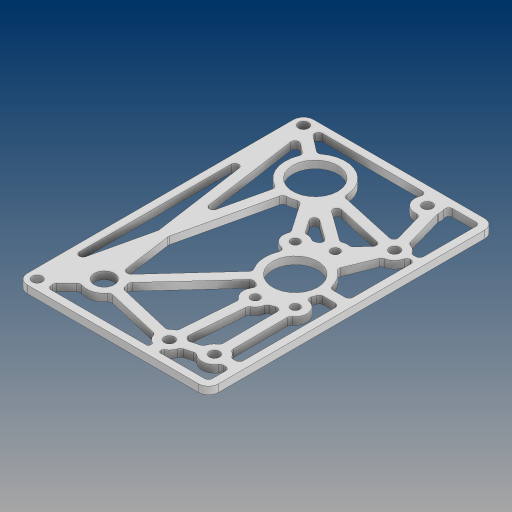
# Autodesk Inventor part: DragBarLinkage3 Bracket1
Saved by Autodesk Inventor 2024.3 (Build 283343000, 343)
## iProperties
Created: 2024-07-08
Part Number: DragBarLinkage3 Bracket1
Material: Generic
Document SubType Name: Modeling
Designer: Kenji
Density: 1 g/cm^3
Appearance: Default
Author: Kenji
Autodesk Inventor part; units mm, degrees
ref_plane "YZ Plane" through (0, 0, 0) normal (1, 0, 0) x (0, 1, 0)
ref_plane "XZ Plane" through (0, 0, 0) normal (0, 1, 0) x (-1, 0, 0)
ref_plane "XY Plane" through (0, 0, 0) normal (0, 0, 1) x (1, 0, 0)
sketch "Sketch1" plane through (0, 0, 0) normal (0, 1, 0) x (-1, 0, 0)
  circle A0 centre (-11.6078, -122.2341) radius 14.2875
  circle A1 centre (0, 0) radius 6.35
  line L0 (-88.9331, 22.86) -> (-88.9331, -149.2216) construction
  circle A2 centre (-11.6078, -122.2341) radius 26.9875 construction
  circle A3 centre (0, 0) radius 19.05 construction
  circle A4 centre (-53.9779, 12.7) radius 3.2512
  circle A5 centre (-62.1078, -142.8716) radius 3.2512
  circle A6 centre (-53.9779, 12.7) radius 6.35 construction
  circle A7 centre (-62.1078, -142.8716) radius 6.35 construction
  line L1 (-56.2297, -140.4694) -> (-36.5897, -132.4433) construction
  line L2 (-68.287, -144.3343) -> (-88.9331, -149.2216) construction
  line L3 (-47.7967, 11.2457) -> (-18.5436, 4.363) construction
  line L4 (-60.0756, 14.4723) -> (-88.9331, 22.86) construction
  line L5 (-88.9331, -32.1945) -> (-26.9571, -32.1945) construction
  line L6 (-26.9571, -32.1945) -> (-26.9571, -94.1705) construction
  line L7 (-26.9571, -94.1705) -> (-88.9331, -94.1705) construction
  line L8 (-88.9331, -94.1705) -> (-88.9331, -32.1945) construction
  circle A8 centre (-57.9451, -63.1825) radius 25.4 construction
  circle A9 centre (-57.9451, -88.5825) radius 2.794
  circle A10 centre (-39.9846, -81.143) radius 2.794
  circle A11 centre (-32.5451, -63.1825) radius 2.794 construction
  circle A12 centre (-39.9846, -45.222) radius 2.794 construction
  circle A13 centre (-57.9451, -37.7825) radius 2.794
  circle A14 centre (-75.9057, -45.222) radius 2.794
  circle A15 centre (-83.3451, -63.1825) radius 2.794 construction
  circle A16 centre (-75.9057, -81.143) radius 2.794 construction
  circle A17 centre (-57.9451, -63.1825) radius 14.2875
  circle A18 centre (-57.9451, -63.1825) radius 22.86 construction
  circle A19 centre (0, 0) radius 22.86 construction
  line L9 (-88.9331, 22.86) -> (22.86, 22.86) construction
  line L10 (22.86, 22.86) -> (22.86, -149.2216) construction
  line L11 (-88.9331, -149.2216) -> (22.86, -149.2216) construction
  line L12 (-93.7083, -147.6341) -> (-93.7083, 21.2725)
  circle A20 centre (21.2725, 21.2725) radius 3.2512
  circle A21 centre (21.2725, 21.2725) radius 6.35 construction
  circle A22 centre (21.2725, -147.6341) radius 3.2512
  circle A23 centre (21.2725, -147.6341) radius 6.35 construction
  line L13 (16.2473, -143.7521) -> (9.7494, -138.7325) construction
  line L14 (16.7824, 16.7824) -> (16.1645, 16.1645) construction
  line L15 (27.6225, 21.2725) -> (27.6225, -147.6341)
  line L16 (21.2725, -153.9841) -> (-87.3583, -153.9841)
  line L17 (21.2725, 27.6225) -> (-87.3583, 27.6225)
  arc A24 (27.6225, 21.2725) -> (21.2725, 27.6225) centre (21.2725, 21.2725) ccw
  arc A25 (21.2725, -153.9841) -> (27.6225, -147.6341) centre (21.2725, -147.6341) ccw
  arc A26 (-87.3583, 27.6225) -> (-93.7083, 21.2725) centre (-87.3583, 21.2725) ccw
  arc A27 (-93.7083, -147.6341) -> (-87.3583, -153.9841) centre (-87.3583, -147.6341) ccw
  circle A28 centre (-76.2331, -107.95) radius 3.2512
  circle A29 centre (-76.2331, 6.35) radius 3.2512
  line L18 (-11.6078, -122.2341) -> (-11.6078, 16.1596) construction
  line L19 (-11.6078, 0) -> (0, 0) construction
  circle A30 centre (-57.9451, -63.1825) radius 19.9136 construction
  circle A31 centre (-11.6078, -122.2341) radius 19.9136 construction
  line L20 (-73.6113, -75.4757) -> (-27.274, -134.5272) construction
  point P0 (0, 19.05)
  point P1 (-11.6078, -149.2216)
  point P2 (-62.1078, -149.2216)
  point P3 (-53.9779, 19.05)
  point P4 (-26.9571, -63.1825)
  point P5 (-57.9451, -32.1945)
  point P6 (0, -63.1825)
  point P7 (0, 22.86)
  point P8 (-93.7083, 27.6225)
  point P9 (-93.7083, -153.9841)
  point P10 (-33.0429, 27.6225)
  point P11 (22.86, -63.1825)
  point P12 (-53.9779, 6.35)
  dimension "d19" = 50.8
  dimension "d289" = 39.8272
  dimension "d290" = 39.8272
  dimension "d1" = 28.575
  dimension "d2" = 12.7
  dimension "d4" = 12.7
  dimension "d5" = 12.7
  dimension "d6" = 6.5024
  dimension "d7" = 6.5024
  dimension "d8" = 12.7
  dimension "d9" = 12.7
  dimension "d17" = 61.976
  dimension "d18" = 61.976
  dimension "d20" = 5.588
  dimension "d23" = 360
  dimension "d25" = 28.575
  dimension "d26" = 45.72
  dimension "d27" = 45.72
  dimension "d31" = 4.7752
  dimension "d32" = 6.5024
  dimension "d33" = 12.7
  dimension "d34" = 6.5024
  dimension "d35" = 12.7
  dimension "d38" = 4.7625
  dimension "d39" = 4.7625
  dimension "d40" = 4.7625
  dimension "d41" = 6.35
  dimension "d42" = 6.35
  dimension "d134" = 6.5024
  dimension "d135" = 6.5024
  dimension "d136" = 12.7
  dimension "d162" = 11.6078
  dimension "d163" = 86.0425
  dimension "d165" = 172.0816
  dimension "d166" = 15.3493
  dimension "d167" = 114.3
  constraints: 44 end point, 29 centre point, 28 point on circle, 18 point on line, 11 tangent, 11 vertical alignment, 10 coincident, 8 horizontal alignment, 5 perpendicular, 3 concentric, 3 horizontal, 3 midpoint, 2 equal length, 2 parallel, 1 collinear, 1 vertical, 28 other
  measures "d1" diameter of A0
  measures "d2" diameter of A1
  measures "d4" radial gap between concentric circles of A0 A2
  measures "d5" radial gap between concentric circles of A1 A3
  measures "d6" diameter of A4
  measures "d7" diameter of A5
  measures "d8" diameter of A6
  measures "d9" diameter of A7
  measures "d17" distance of L6.end L7.end
  measures "d18" distance of L5.end L6.end
  measures "d20" diameter of A9
  measures "d25" diameter of A17
  measures "d26" diameter of A18
  measures "d27" diameter of A19
  measures "d31" distance between parallel lines of L12 L0
  measures "d32" diameter of A20
  measures "d33" diameter of A21
  measures "d34" diameter of A22
  measures "d35" diameter of A23
  measures "d38" distance between parallel lines of L10 L15
  measures "d39" distance between parallel lines of L16 L11
  measures "d40" distance from line of point (-33.043, 27.623) L9
  measures "d41" radius of A26
  measures "d42" radius of A27
  measures "d134" diameter of A28
  measures "d135" diameter of A29
  measures "d136" distance from line of L0 A29.centre
  measures "d162" distance of L19.start L19.end
  measures "d163" distance of L9.end point (22.86, -63.183)
  measures "d165" distance of L9.end L10.end
  measures "d166" distance between parallel lines of L6 L18
  measures "d167" distance of A28.centre A29.centre
extrude "Extrusion2" add sketch "Sketch1" along normal blind 4.7625 contours L12 A26 L17 A24 L15 A25 L16 A27 | A28 | A29
extrude "Extrusion5" cut sketch "Sketch1" along normal blind 25.4 contours A28 | A29
sketch "Sketch6" plane through (0, 4.7625, 0) normal (0, 1, 0) x (1, 0, 0)
  circle A0 centre (76.2331, -6.35) radius 3.2512 projected
  circle A1 centre (76.2331, 107.95) radius 3.2512 projected
  line L0 (-27.6225, 147.6341) -> (-27.6225, -21.2725) projected
  arc A2 (-27.6225, -21.2725) -> (-21.2725, -27.6225) centre (-21.2725, -21.2725) ccw projected
  line L1 (-21.2725, -27.6225) -> (87.3583, -27.6225) projected
  arc A3 (87.3583, -27.6225) -> (93.7083, -21.2725) centre (87.3583, -21.2725) ccw projected
  line L2 (93.7083, -21.2725) -> (93.7083, 147.6341) projected
  arc A4 (93.7083, 147.6341) -> (87.3583, 153.9841) centre (87.3583, 147.6341) ccw projected
  line L3 (87.3583, 153.9841) -> (-21.2725, 153.9841) projected
  arc A5 (-21.2725, 153.9841) -> (-27.6225, 147.6341) centre (-21.2725, 147.6341) ccw projected
  circle A6 centre (57.9451, 63.1825) radius 14.2875 projected
  circle A7 centre (11.6078, 122.2341) radius 14.2875 projected
  circle A8 centre (0, 0) radius 6.35 projected
  circle A9 centre (53.9779, -12.7) radius 3.2512 projected
  circle A10 centre (62.1078, 142.8716) radius 3.2512 projected
  circle A11 centre (57.9451, 88.5825) radius 2.794 projected
  circle A12 centre (39.9846, 81.143) radius 2.794 projected
  circle A13 centre (57.9451, 37.7825) radius 2.794 projected
  circle A14 centre (75.9057, 45.222) radius 2.794 projected
  circle A15 centre (-21.2725, 147.6341) radius 3.2512 projected
  circle A16 centre (-21.2725, -21.2725) radius 3.2512 projected
  circle A17 centre (0, 0) radius 11.1252 construction
  circle A18 centre (-21.2725, -21.2725) radius 8.0137 construction
  circle A19 centre (11.6078, 122.2341) radius 19.05 construction
  circle A20 centre (57.9451, 63.1825) radius 19.05 construction
  circle A21 centre (39.9846, 81.143) radius 7.5565 construction
  circle A22 centre (57.9451, 37.7825) radius 7.5565 construction
  circle A23 centre (75.9057, 45.222) radius 7.5565 construction
  circle A24 centre (57.9451, 88.5825) radius 7.5565 construction
  circle A25 centre (76.2331, 107.95) radius 8.0137 construction
  circle A26 centre (62.1078, 142.8716) radius 8.0137 construction
  circle A27 centre (-21.2725, 147.6341) radius 8.0137 construction
  circle A28 centre (53.9779, -12.7) radius 8.0137 construction
  circle A29 centre (76.2331, -6.35) radius 8.0137 construction
  line L4 (-15.606, -15.606) -> (-7.8667, -7.8667) construction
  line L5 (7.5195, 8.1992) -> (45.0692, 49.1428) construction
  line L6 (35.6906, 87.3609) -> (22.433, 106.5587) construction
  line L7 (-3.4678, 133.88) -> (-14.9307, 142.735) construction
  line L8 (27.0219, 111.0399) -> (51.8309, 93.0228) construction
  line L9 (57.3531, 30.2492) -> (54.6057, -4.7109) construction
  line L10 (46.1772, -10.8646) -> (10.8295, -2.548) construction
  line L11 (61.6841, -10.5012) -> (68.527, -8.5488) construction
  line L12 (76.1823, 1.6635) -> (75.9536, 37.6656) construction
  line L13 (63.1331, 94.0767) -> (70.7313, 102.1234) construction
  line L14 (73.2026, 100.5314) -> (65.1493, 80.8178) construction
  line L15 (68.4083, 109.6795) -> (30.2089, 118.1227) construction
  line L16 (74.0344, 115.6562) -> (67.8609, 137.2929) construction
  line L17 (-22.8473, -21.2725) -> (-22.8473, 147.6341) construction
  arc A30 (-21.2725, 149.2089) -> (-22.8473, 147.6341) centre (-21.2725, 147.6341) ccw construction
  line L18 (-10.9265, 149.2089) -> (86.5709, 149.2089) construction
  arc A31 (88.9331, 147.6341) -> (87.3583, 149.2089) centre (87.3583, 147.6341) ccw construction
  line L19 (88.9331, -11.8872) -> (88.9331, -21.2725) construction
  arc A32 (87.3583, -22.8473) -> (88.9331, -21.2725) centre (87.3583, -21.2725) ccw construction
  line L20 (87.3583, -22.8473) -> (-10.9265, -22.8473) construction
  arc A33 (-22.8473, -21.2725) -> (-21.2725, -22.8473) centre (-21.2725, -21.2725) ccw construction
  line L21 (76.9951, 63.1825) -> (88.9331, 63.1825) construction
  line L22 (46.9659, 84.0348) -> (50.9638, 85.6908) construction
  line L23 (64.9264, 40.6742) -> (68.9244, 42.3302) construction
  line L24 (-19.4828, -13.4612) -> (7.3533, 103.6652) construction
  line L25 (-20.1296, 139.7023) -> (-6.3312, 43.9392) construction
  line L26 (-18.1826, 6.43) -> (-9.6563, 43.6428)
  line L27 (-18.147, 103.6805) -> (-9.6208, 44.5073)
  line L28 (-22.8473, 6.9575) -> (-22.8473, 103.3436)
  arc A34 (-22.8473, 6.9575) -> (-18.1826, 6.43) centre (-20.4851, 6.9575) ccw
  arc A35 (-18.147, 103.6805) -> (-22.8473, 103.3436) centre (-20.4851, 103.3436) ccw
  arc A36 (-9.6563, 43.6428) -> (-9.6208, 44.5073) centre (-11.9589, 44.1704) ccw
  line L29 (-16.181, 134.5609) -> (-7.4279, 73.8134)
  line L30 (-3.006, 44.2355) -> (10.0832, 101.3636)
  line L31 (-2.7873, 73.6227) -> (3.8936, 102.7817)
  line L32 (-6.7018, 132.3662) -> (-12.3989, 136.7672)
  line L33 (-6.3312, 43.9392) -> (-1.5866, 11.0115) construction
  line L34 (1.3886, 12.6254) -> (-3.0415, 43.3711)
  line L35 (5.9725, 11.2098) -> (41.625, 50.0846)
  line L36 (32.6958, 86.1103) -> (20.7488, 103.4101)
  arc A37 (12.2999, 103.1967) -> (18.0111, 104.2925) centre (11.6078, 122.2341) ccw
  arc A38 (32.9509, 83.9046) -> (38.6015, 73.7142) centre (39.9846, 81.143) ccw
  arc A39 (40.3509, 70.4862) -> (41.8765, 52.9501) centre (57.9451, 63.1825) ccw
  arc A40 (3.4905, 10.5635) -> (3.074, 10.6921) centre (0, 0) ccw
  arc A41 (1.3886, 12.6254) -> (3.074, 10.6921) centre (3.7267, 12.9623) ccw
  arc A42 (3.4905, 10.5635) -> (5.9725, 11.2098) centre (4.2316, 12.8064) ccw
  arc A43 (-3.006, 44.2355) -> (-3.0415, 43.3711) centre (-0.7035, 43.7079) ccw
  arc A44 (41.625, 50.0846) -> (41.8765, 52.9501) centre (39.884, 51.6813) ccw
  arc A45 (40.3509, 70.4862) -> (38.6015, 73.7142) centre (38.1692, 71.3919) ccw
  arc A46 (32.9509, 83.9046) -> (32.6958, 86.1103) centre (30.7521, 84.768) ccw
  arc A47 (20.7488, 103.4101) -> (18.0111, 104.2925) centre (18.8051, 102.0677) ccw
  arc A48 (12.2999, 103.1967) -> (10.0832, 101.3636) centre (12.3857, 100.836) ccw
  arc A49 (-7.4279, 73.8134) -> (-2.7873, 73.6227) centre (-5.0899, 74.1502) ccw
  arc A50 (-12.3989, 136.7672) -> (-16.181, 134.5609) centre (-13.843, 134.8978) ccw
  arc A51 (-5.9667, 129.5853) -> (2.6961, 105.3971) centre (11.6078, 122.2341) ccw
  arc A52 (3.8936, 102.7817) -> (2.6961, 105.3971) centre (1.5911, 103.3093) ccw
  arc A53 (-5.9667, 129.5853) -> (-6.7018, 132.3662) centre (-8.1459, 130.4968) ccw
  line L37 (-12.8227, -17.3128) -> (-6.4512, -10.9413)
  line L38 (44.7091, -13.7809) -> (11.2443, -5.9073)
  line L39 (53.9779, -20.7137) -> (53.9779, -22.8473) construction
  line L40 (84.2468, -6.35) -> (88.9331, -6.35) construction
  line L41 (-13.4151, -22.8473) -> (49.6218, -22.8473)
  arc A54 (46.4014, -15.3108) -> (50.1814, -19.7573) centre (53.9779, -12.7) ccw
  arc A55 (-3.9435, -10.4028) -> (8.8287, -6.7694) centre (0, 0) ccw
  arc A56 (-13.2819, -20.6644) -> (-13.4563, -19.5043) centre (-21.2725, -21.2725) ccw
  arc A57 (-12.8227, -17.3128) -> (-13.4563, -19.5043) centre (-11.1523, -18.9831) ccw
  arc A58 (-13.2819, -20.6644) -> (-10.9265, -22.8473) centre (-10.9265, -20.4851) ccw
  arc A59 (-3.9435, -10.4028) -> (-6.4512, -10.9413) centre (-4.7809, -12.6116) ccw
  arc A60 (11.2443, -5.9073) -> (8.8287, -6.7694) centre (10.7033, -8.2067) ccw
  arc A61 (46.4014, -15.3108) -> (44.7091, -13.7809) centre (44.1681, -16.0803) ccw
  circle A62 centre (49.6218, -21.6662) radius 1.1811 construction
  arc A63 (48.5235, -21.2318) -> (50.7201, -21.2318) centre (49.6218, -20.7975) ccw construction
  line L42 (50.8029, -20.7975) -> (50.8029, -21.6662)
  arc A64 (50.8029, -20.7975) -> (50.1814, -19.7573) centre (49.6218, -20.7975) ccw construction
  arc A65 (49.6218, -22.8473) -> (50.8029, -21.6662) centre (49.6218, -21.6662) ccw
  arc A66 (50.8029, -20.7975) -> (50.1814, -19.7573) centre (49.6218, -20.7975) ccw
  line L43 (46.1634, -7.5997) -> (12.6986, 0.2739)
  line L44 (10.6524, 6.9178) -> (46.3049, 45.7927)
  line L45 (54.1352, 29.8273) -> (51.5001, -3.7033)
  arc A67 (50.2454, -5.6086) -> (48.3603, -6.9849) centre (53.9779, -12.7) ccw
  arc A68 (49.1379, 46.2907) -> (50.6686, 45.577) centre (57.9451, 63.1825) ccw
  arc A69 (51.7142, 42.0575) -> (53.2485, 31.8629) centre (57.9451, 37.7825) ccw
  arc A70 (10.9208, 2.1227) -> (10.2228, 4.3892) centre (0, 0) ccw
  arc A71 (10.6524, 6.9178) -> (10.2228, 4.3892) centre (12.3933, 5.3212) ccw
  arc A72 (10.9208, 2.1227) -> (12.6986, 0.2739) centre (13.2396, 2.5734) ccw
  arc A73 (46.1634, -7.5997) -> (48.3603, -6.9849) centre (46.7044, -5.3003) ccw
  arc A74 (50.2454, -5.6086) -> (51.5001, -3.7033) centre (49.1452, -3.5183) ccw
  arc A75 (49.1379, 46.2907) -> (46.3049, 45.7927) centre (48.0458, 44.1961) ccw
  arc A76 (51.7142, 42.0575) -> (50.6686, 45.577) centre (49.7663, 43.3939) ccw
  arc A77 (54.1352, 29.8273) -> (53.2485, 31.8629) centre (51.7802, 30.0124) ccw
  line L46 (37.9209, 89.7187) -> (32.6443, 97.3594)
  line L47 (35.9762, 100.6131) -> (48.0773, 91.8249)
  line L48 (46.3724, 87.2255) -> (47.5932, 87.7312)
  arc A78 (35.9762, 100.6131) -> (32.6443, 97.3594) centre (34.5881, 98.7018) ccw
  arc A79 (50.5311, 90.0429) -> (50.395, 88.8917) centre (57.9451, 88.5825) ccw
  arc A80 (44.1624, 87.4396) -> (39.8933, 88.699) centre (39.9846, 81.143) ccw
  arc A81 (37.9209, 89.7187) -> (39.8933, 88.699) centre (39.8647, 91.061) ccw
  arc A82 (44.1624, 87.4396) -> (46.3724, 87.2255) centre (45.4684, 89.4079) ccw
  arc A83 (47.5932, 87.7312) -> (48.0773, 91.8249) centre (46.6892, 89.9136) ccw
  line L49 (60.4657, 29.3298) -> (57.8306, -4.2008)
  line L50 (61.5449, -7.2392) -> (66.9239, -5.7045)
  line L51 (73.0025, 2.4046) -> (72.783, 36.9717)
  line L52 (66.763, 37.9984) -> (69.5169, 39.1391)
  arc A84 (59.3216, -6.728) -> (58.7723, -6.2787) centre (53.9779, -12.7) ccw
  arc A85 (61.6595, 31.2019) -> (65.3516, 36.2843) centre (57.9451, 37.7825) ccw
  arc A86 (70.7855, 39.6646) -> (72.7743, 38.3448) centre (75.9057, 45.222) ccw
  arc A87 (71.9136, 0.3999) -> (68.5427, -4.097) centre (76.2331, -6.35) ccw
  arc A88 (57.8306, -4.2008) -> (58.7723, -6.2787) centre (60.1856, -4.3859) ccw
  arc A89 (59.3216, -6.728) -> (61.5449, -7.2392) centre (60.8968, -4.9677) ccw
  arc A90 (61.6595, 31.2019) -> (60.4657, 29.3298) centre (62.8206, 29.1448) ccw
  arc A91 (66.763, 37.9984) -> (65.3516, 36.2843) centre (67.6669, 35.816) ccw
  arc A92 (72.783, 36.9717) -> (69.5169, 39.1391) centre (70.4208, 36.9567) ccw
  arc A93 (66.9239, -5.7045) -> (68.5427, -4.097) centre (66.2757, -3.4329) ccw
  arc A94 (71.9136, 0.3999) -> (73.0025, 2.4046) centre (70.6403, 2.3896) ccw
  line L53 (63.2872, -13.3455) -> (68.6662, -11.8108)
  line L54 (85.008, -9.525) -> (86.5709, -9.525)
  line L55 (88.9331, -9.525) -> (88.9331, -20.4851)
  arc A95 (70.8894, -12.322) -> (83.0103, -10.6266) centre (76.2331, -6.35) ccw
  arc A96 (63.2872, -13.3455) -> (61.6684, -14.953) centre (63.9353, -15.6171) ccw
  arc A97 (70.8894, -12.322) -> (68.6662, -11.8108) centre (69.3143, -14.0823) ccw
  arc A98 (85.008, -9.525) -> (83.0103, -10.6266) centre (85.008, -11.8872) ccw
  arc A99 (88.9331, -11.8872) -> (86.5709, -9.525) centre (86.5709, -11.8872) ccw
  arc A100 (86.5709, -22.8473) -> (88.9331, -20.4851) centre (86.5709, -20.4851) ccw
  circle A101 centre (58.334, -20.7975) radius 1.1811 construction
  circle A102 centre (58.334, -21.6662) radius 1.1811 construction
  line L56 (57.1529, -20.7975) -> (57.1529, -21.6662)
  arc A103 (57.7745, -19.7573) -> (61.6684, -14.953) centre (53.9779, -12.7) ccw
  line L57 (58.334, -22.8473) -> (86.5709, -22.8473)
  arc A104 (57.1529, -21.6662) -> (58.334, -22.8473) centre (58.334, -21.6662) ccw
  arc A105 (57.7745, -19.7573) -> (57.1529, -20.7975) centre (58.334, -20.7975) ccw
  line L58 (85.008, -3.175) -> (86.5709, -3.175)
  line L59 (79.3524, 2.4449) -> (79.1328, 37.0131)
  line L60 (78.629, 60.0075) -> (86.5709, 60.0075)
  line L61 (88.9331, -0.8128) -> (88.9331, 57.6453)
  arc A106 (80.1639, 38.9795) -> (77.2887, 52.6508) centre (75.9057, 45.222) ccw
  arc A107 (75.5394, 55.8788) -> (76.3471, 58.2562) centre (57.9451, 63.1825) ccw
  arc A108 (83.0103, -2.0734) -> (80.4666, 0.4542) centre (76.2331, -6.35) ccw
  arc A109 (79.3524, 2.4449) -> (80.4666, 0.4542) centre (81.7145, 2.4599) ccw
  arc A110 (83.0103, -2.0734) -> (85.008, -3.175) centre (85.008, -0.8128) ccw
  arc A111 (86.5709, -3.175) -> (88.9331, -0.8128) centre (86.5709, -0.8128) ccw
  arc A112 (80.1639, 38.9795) -> (79.1328, 37.0131) centre (81.495, 37.0281) ccw
  arc A113 (75.5394, 55.8788) -> (77.2887, 52.6508) centre (77.7211, 54.9731) ccw
  arc A114 (78.629, 60.0075) -> (76.3471, 58.2562) centre (78.629, 57.6453) ccw
  arc A115 (88.9331, 57.6453) -> (86.5709, 60.0075) centre (86.5709, 57.6453) ccw
  line L62 (75.8539, 98.6261) -> (68.7064, 81.1296)
  line L63 (78.629, 66.3575) -> (86.5709, 66.3575)
  line L64 (76.8787, 117.2593) -> (70.1293, 140.9144)
  line L65 (84.2468, 107.95) -> (93.7083, 107.95) construction
  line L66 (88.9331, 68.7197) -> (88.9331, 105.5878)
  line L67 (86.3366, 107.95) -> (86.5709, 107.95)
  arc A116 (77.6292, 100.0588) -> (84.0364, 106.1256) centre (76.2331, 107.95) ccw
  arc A117 (76.3471, 68.1088) -> (69.4648, 78.3549) centre (57.9451, 63.1825) ccw
  arc A118 (68.7064, 81.1296) -> (69.4648, 78.3549) centre (70.8932, 80.2362) ccw
  arc A119 (76.3471, 68.1088) -> (78.629, 66.3575) centre (78.629, 68.7197) ccw
  arc A120 (86.5709, 66.3575) -> (88.9331, 68.7197) centre (86.5709, 68.7197) ccw
  arc A121 (77.6292, 100.0588) -> (75.8539, 98.6261) centre (78.0407, 97.7328) ccw
  arc A122 (86.3366, 107.95) -> (84.0364, 106.1256) centre (86.3366, 105.5878) ccw
  arc A123 (88.9331, 105.5878) -> (86.5709, 107.95) centre (86.5709, 105.5878) ccw
  line L68 (85.008, 111.125) -> (86.5709, 111.125)
  line L69 (88.9331, 113.4872) -> (88.9331, 146.8467)
  arc A124 (83.0103, 112.2266) -> (78.4861, 115.6405) centre (76.2331, 107.95) ccw
  arc A125 (70.0575, 141.8605) -> (69.5101, 145.9417) centre (62.1078, 142.8716) ccw
  line L70 (71.6921, 149.2089) -> (88.9331, 149.2089)
  arc A126 (76.8787, 117.2593) -> (78.4861, 115.6405) centre (79.1502, 117.9074) ccw
  arc A127 (83.0103, 112.2266) -> (85.008, 111.125) centre (85.008, 113.4872) ccw
  arc A128 (86.5709, 111.125) -> (88.9331, 113.4872) centre (86.5709, 113.4872) ccw
  arc A129 (88.9331, 146.8467) -> (86.5709, 149.2089) centre (86.5709, 146.8467) ccw
  arc A130 (71.6921, 149.2089) -> (69.5101, 145.9417) centre (71.6921, 146.8467) ccw
  arc A131 (70.0575, 141.8605) -> (70.1293, 140.9144) centre (72.4008, 141.5625) ccw
  line L71 (34.9904, 109.1768) -> (53.1523, 95.9872)
  line L72 (66.0121, 106.9575) -> (36.8883, 113.3947)
  line L73 (61.2865, 96.7456) -> (67.2198, 103.0292)
  arc A132 (28.672, 113.7655) -> (29.2635, 115.08) centre (11.6078, 122.2341) ccw
  arc A133 (59.1822, 96.037) -> (55.3512, 95.6798) centre (57.9451, 88.5825) ccw
  arc A134 (68.3634, 106.4378) -> (68.8731, 104.78) centre (76.2331, 107.95) ccw
  arc A135 (36.8883, 113.3947) -> (34.9904, 109.1768) centre (36.3785, 111.0882) ccw
  arc A136 (53.1523, 95.9872) -> (55.3512, 95.6798) centre (54.5403, 97.8985) ccw
  arc A137 (59.1822, 96.037) -> (61.2865, 96.7456) centre (59.569, 98.3674) ccw
  arc A138 (67.2198, 103.0292) -> (66.0121, 106.9575) centre (65.5023, 104.651) ccw
  line L74 (-2.8198, 137.3914) -> (-12.3873, 144.7823)
  line L75 (67.8506, 113.0544) -> (32.4894, 120.8703)
  line L76 (70.632, 116.0091) -> (65.7182, 133.2306)
  line L77 (-13.4151, 149.2089) -> (52.5236, 149.2089)
  arc A139 (30.6393, 123.0728) -> (0.0566, 137.3824) centre (11.6078, 122.2341) ccw
  arc A140 (-13.2948, 146.8753) -> (-13.2819, 147.0259) centre (-21.2725, 147.6341) ccw
  arc A141 (54.7055, 145.9417) -> (63.1419, 134.9249) centre (62.1078, 142.8716) ccw
  arc A142 (71.1612, 114.1544) -> (69.7339, 112.6382) centre (76.2331, 107.95) ccw
  arc A143 (-13.2948, 146.8753) -> (-12.3873, 144.7823) centre (-10.9432, 146.6517) ccw
  arc A144 (-10.9265, 149.2089) -> (-13.2819, 147.0259) centre (-10.9265, 146.8467) ccw
  arc A145 (-2.8198, 137.3914) -> (0.0566, 137.3824) centre (-1.3757, 139.2608) ccw
  arc A146 (30.6393, 123.0728) -> (32.4894, 120.8703) centre (32.9992, 123.1768) ccw
  arc A147 (67.8506, 113.0544) -> (70.632, 116.0091) centre (68.3604, 115.3609) ccw
  arc A148 (65.7182, 133.2306) -> (63.1419, 134.9249) centre (63.4467, 132.5824) ccw
  arc A149 (54.7055, 145.9417) -> (52.5236, 149.2089) centre (52.5236, 146.8467) ccw
  point P0 (-22.8473, 63.1808)
  point P1 (-22.724, -13.3914)
  point P2 (-22.8473, 136.3009)
  point P3 (-22.8473, -13.4151)
  point P4 (-3.1043, 43.8066)
  point P5 (10.5076, 103.2159)
  point P6 (4.318, 104.634)
  point P7 (-5.198, 131.2045)
  point P8 (1.6219, 11.0063)
  point P9 (4.8669, 10.0042)
  point P10 (42.9094, 51.4852)
  point P11 (33.4755, 84.9812)
  point P12 (19.669, 104.9737)
  point P13 (-13.8246, -18.3147)
  point P14 (-5.2945, -9.7846)
  point P15 (46.0884, -14.1054)
  point P16 (9.652, -5.5326)
  point P17 (47.5428, -7.9242)
  point P18 (11.1063, 0.6486)
  point P19 (9.5468, 5.7122)
  point P20 (47.5893, 47.1932)
  point P21 (54.2427, 31.1952)
  point P22 (51.3891, -5.116)
  point P23 (38.7006, 88.5896)
  point P24 (24.8941, 108.5821)
  point P25 (24.9406, 108.6275)
  point P26 (45.1048, 86.7004)
  point P27 (60.5732, 30.6977)
  point P28 (57.7196, -5.6135)
  point P29 (60.1823, -7.628)
  point P30 (68.2865, -5.3157)
  point P31 (73.0115, 0.9876)
  point P32 (65.4953, 37.4733)
  point P33 (61.9246, -13.7343)
  point P34 (70.0288, -11.422)
  point P35 (83.591, -9.525)
  point P36 (83.591, -3.175)
  point P37 (79.3614, 1.0279)
  point P38 (79.1241, 38.3852)
  point P39 (76.7287, 60.0075)
  point P40 (76.3898, 99.9378)
  point P41 (67.9878, 79.3704)
  point P42 (76.7287, 66.3575)
  point P43 (77.2675, 115.8967)
  point P44 (69.9874, 141.4116)
  point P45 (88.9331, 107.95)
  point P46 (83.591, 111.125)
  point P47 (67.0127, 149.2089)
  point P48 (54.2625, 95.1809)
  point P49 (60.3444, 95.748)
  point P50 (-1.316, 136.2297)
  point P51 (-13.5087, 145.6485)
  point P52 (30.6339, 121.2804)
  point P53 (65.0897, 135.4333)
  point P54 (57.2029, 149.2089)
  point P55 (57.7745, -19.7573)
  dimension "d199" = 4.7752
  dimension "d200" = 4.7625
  dimension "d201" = 4.7625
  dimension "d202" = 4.7625
  dimension "d203" = 4.7625
  dimension "d204" = 4.7752
  dimension "d205" = 4.7752
  dimension "d206" = 4.7752
  dimension "d207" = 4.7752
  dimension "d208" = 4.7752
  dimension "d209" = 3.175
  dimension "d210" = 3.175
  dimension "d211" = 2.3622
  dimension "d212" = 2.3622
  dimension "d213" = 2.3622
  dimension "d217" = 3.175
  dimension "d218" = 3.175
  dimension "d219" = 3.175
  dimension "d220" = 3.175
  dimension "d223" = 3.175
  dimension "d224" = 3.175
  dimension "d225" = 3.175
  dimension "d226" = 2.3622
  dimension "d227" = 2.3622
  dimension "d228" = 2.3622
  dimension "d229" = 2.3622
  dimension "d230" = 3.175
  dimension "d231" = 3.175
  dimension "d233" = 2.3622
  dimension "d234" = 2.3622
  dimension "d235" = 2.3622
  dimension "d236" = 3.175
  dimension "d237" = 3.175
  dimension "d238" = 3.175
  dimension "d239" = 3.175
  dimension "d240" = 2.3622
  dimension "d241" = 3.175
  dimension "d243" = 3.175
  dimension "d244" = 3.175
  dimension "d245" = 2.3622
  dimension "d246" = 2.3622
  dimension "d247" = 3.175
  dimension "d248" = 3.175
  dimension "d249" = 3.175
  dimension "d250" = 3.175
  dimension "d251" = 2.3622
  dimension "d252" = 2.3622
  dimension "d253" = 2.3622
  dimension "d254" = 3.175
  dimension "d256" = 3.175
  dimension "d257" = 2.3622
  dimension "d258" = 2.3622
  dimension "d259" = 2.3622
  dimension "d260" = 2.3622
  dimension "d261" = 3.175
  dimension "d262" = 4.7625
  dimension "d263" = 3.175
  dimension "d264" = 3.175
  dimension "d265" = 3.175
  dimension "d266" = 4.7752
  dimension "d267" = 2.3622
  dimension "d268" = 2.3622
  dimension "d269" = 3.175
  dimension "d270" = 3.175
  constraints: 321 point on circle, 156 tangent, 148 end point, 126 centre point, 126 point on line, 54 equal radius, 16 concentric, 8 parallel, 5 collinear, 5 perpendicular, 2 horizontal alignment, 2 vertical, 2 vertical alignment, 1 coincident, 1 horizontal, 1 midpoint, 119 other
  measures "d200" radial gap between concentric circles of A16 A18
  measures "d204" distance between parallel lines of L18 L3
  measures "d205" distance between parallel lines of L17 L0
  measures "d206" distance between parallel lines of L1 L20
  measures "d207" distance between parallel lines of L2 L19
  measures "d208" distance of L2.start L19.end
  measures "d209" distance between parallel lines of L25 L27
  measures "d210" distance between parallel lines of L24 L26
  measures "d211" radius of A34
  measures "d212" radius of A35
  measures "d213" radius of A36
  measures "d217" distance between parallel lines of L29 L25
  measures "d218" distance between parallel lines of L7 L32
  measures "d219" distance between parallel lines of L24 L31
  measures "d220" distance between parallel lines of L30 L24
  measures "d223" distance between parallel lines of L34 L33
  measures "d224" distance between parallel lines of L5 L35
  measures "d225" distance between parallel lines of L6 L36
  measures "d226" radius of A41
  measures "d227" radius of A43
  measures "d228" radius of A49
  measures "d229" radius of A52
  measures "d230" distance between parallel lines of L10 L38
  measures "d231" distance between parallel lines of L37 L4
  measures "d233" radius of A57
  measures "d234" diameter of A62
  measures "d235" diameter of A63
  measures "d236" distance between parallel lines of L39 L42
  measures "d237" distance between parallel lines of L10 L43
  measures "d238" distance between parallel lines of L44 L5
  measures "d239" distance between parallel lines of L9 L45
  measures "d240" radius of A71
  measures "d241" distance between parallel lines of L8 L47
  measures "d243" distance between parallel lines of L22 L48
  measures "d244" distance between parallel lines of L6 L46
  measures "d245" radius of A78
  measures "d246" radius of A81
  measures "d247" distance between parallel lines of L52 L23
  measures "d248" distance between parallel lines of L49 L9
  measures "d249" distance between parallel lines of L11 L50
  measures "d250" distance between parallel lines of L12 L51
  measures "d251" radius of A88
  measures "d252" radius of A92
  measures "d253" radius of A93
  measures "d254" distance between parallel lines of L53 L11
  measures "d256" distance between parallel lines of L40 L54
  measures "d257" radius of A96
  measures "d258" radius of A100
  measures "d259" diameter of A101
  measures "d260" diameter of A102
  measures "d261" distance between parallel lines of L39 L56
  measures "d262" radial gap between concentric circles of A9 A103
  measures "d263" distance between parallel lines of L59 L12
  measures "d264" distance between parallel lines of L40 L58
  measures "d265" distance between parallel lines of L21 L60
  measures "d266" distance between parallel lines of L2 L61
  measures "d267" radius of A109
  measures "d268" radius of A115
  measures "d269" distance between parallel lines of L21 L63
  measures "d270" distance between parallel lines of L14 L62
extrude "Extrusion6" cut sketch "Sketch6" against normal blind 25.4 contours A34 L28 A35 L27 A36 L26 | A50 L32 A53 A51 A52 L31 A49 L29 | L30 A48 A37 A47 L36 A46 A38 A45 A39 A44 L35 A42 A40 A41 L34 A43 | L37 A59 A55 A60 L38 A61 A54 A66 L42 A65 L41 A58 A56 A57 | L43 A72 A70 A71 L44 A75 A68 A76 A69 A77 L45 A74 A67 A73 | L46 A78 L47 A83 L48 A82 A80 A81 | A90 A85 A91 L52 A92 L51 A94 A87 A93 L50 A89 A84 A88 L49 | L53 A97 A95 A98 L54 A99 L55 A100 L57 A104 L56 A105 A103 A96 | A110 A108 A109 L59 A112 A106 A113 A107 A114 L60 A115 L61 A111 L58 | A121 A116 A122 L67 A123 L66 A120 L63 A119 A117 A118 L62 | L64 A131 A125 A130 L70 A129 L69 A128 L68 A127 A124 A126 | A135 L72 A138 L73 A137 A133 A136 L71 | L74 A143 A140 A144 L77 A149 A141 A148 L76 A147 L75 A146 A139 A145
body "Solid2"
